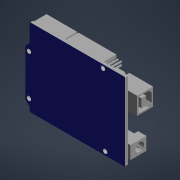
# Autodesk Inventor part: Arduino_Uno
Saved by Autodesk Inventor 2022 (Build 260153000, 153)
## iProperties
Created: 2016-11-21
Part Number: Arduino_Uno
Material: Genérico
Document SubType Name: Modeling
Designer: Dimitris
Density: 1 g/cm^3
Appearance: Por defecto
Author: Dimitris
Autodesk Inventor part; units mm, degrees
ref_plane "YZ Plane" through (0, 0, 0) normal (1, 0, 0) x (0, 1, 0)
ref_plane "XZ Plane" through (0, 0, 0) normal (0, 1, 0) x (-1, 0, 0)
sketch "Sketch1" plane through (0, 0, 0) normal (0, 1, 0) x (-1, 0, 0)
  line L0 (-3.5, 0) -> (-68, 0)
  line L1 (-68.5, -0.5) -> (-68.5, -53)
  line L2 (-68, -53.5) -> (-3.5, -53.5)
  line L3 (-3, -53) -> (-3, -50.5)
  line L4 (-3, -50.5) -> (-0.1464, -47.6464)
  line L5 (0, -15.7071) -> (0, -47.2929)
  line L6 (-3, -0.5) -> (-3, -12.5)
  line L7 (-0.1464, -15.3536) -> (-3, -12.5)
  arc A0 (-68.5, -53) -> (-68, -53.5) centre (-68, -53) ccw
  arc A1 (-68, 0) -> (-68.5, -0.5) centre (-68, -0.5) ccw
  arc A2 (-3.5, -53.5) -> (-3, -53) centre (-3.5, -53) ccw
  arc A3 (-0.1464, -47.6464) -> (0, -47.2929) centre (-0.5, -47.2929) ccw
  arc A4 (0, -15.7071) -> (-0.1464, -15.3536) centre (-0.5, -15.7071) ccw
  arc A5 (-3, -0.5) -> (-3.5, 0) centre (-3.5, -0.5) ccw
  point P0 (0, 0)
  point P1 (-68.5, -53.5)
  point P2 (-68.5, 0)
  point P3 (0, -47.5)
  point P4 (-3, -53.5)
  point P5 (0, -15.5)
  point P6 (-3, 0)
  dimension "d1" = 53.5
  dimension "d3" = 3
  dimension "d5" = 6
  dimension "d6" = 3
  dimension "d7" = 12.5
  dimension "d9" = 65.5
  dimension "d10" = 65.5
  dimension "d11" = 38
  dimension "d12" = 32
  dimension "d13" = 0.5
  constraints: 16 end point, 12 point on circle, 12 point on line, 12 tangent, 6 centre point, 5 equal radius, 3 parallel, 3 perpendicular, 1 horizontal
  measures "d1" distance of point (-68.5, -53.5) point (-68.5, 0)
  measures "d3" distance of point (-3, -53.5) L3.end
  measures "d5" distance from line of point (0, -47.5) L2
  measures "d6" distance between parallel lines of L5 L3
  measures "d7" distance of point (-3, 0) L6.end
  measures "d9" distance between parallel lines of L1 L6
  measures "d10" distance between parallel lines of L1 L3
  measures "d11" distance of L3.end L6.end
  measures "d12" distance of point (0, -15.5) point (0, -47.5)
  measures "d13" radius of A0
extrude "Extrusion1" add sketch "Sketch1" along normal blind 2
sketch "Sketch2" plane through (0, 2, 0) normal (0, 1, 0) x (1, 0, 0)
  line L0 (58.5, 1) -> (64.7, 1)
  line L1 (64.7, 1) -> (64.7, 7.2)
  line L2 (64.7, 7.2) -> (58.5, 7.2)
  line L3 (58.5, 7.2) -> (58.5, 1)
  point P0 (0, 0)
  dimension "d16" = 6.2
  dimension "d17" = 6.2
  constraints: 8 end point, 2 parallel, 1 horizontal, 1 perpendicular
  measures "d16" distance of L2.end L1.end
  measures "d17" distance of L1.end L0.end
extrude "Extrusion2" add sketch "Sketch2" along normal blind 2
sketch "Sketch3" plane through (0, 4, 0) normal (0, 1, 0) x (1, 0, 0)
  circle A0 centre (61.6, 4.1) radius 1.57
  point P0 (0, 0)
  dimension "d20" = 3.14
  constraints: 1 centre point
  measures "d20" diameter of A0
extrude "Extrusion3" add sketch "Sketch3" along normal blind 1.5
sketch "Sketch4" plane through (0, 2, 0) normal (0, 1, 0) x (1, 0, 0)
  line L0 (64.7, 7.2) -> (64.7, 1) projected
  line L1 (64.72, 1) -> (66.7, 1)
  line L2 (66.7, 1) -> (66.7, 1.8)
  line L3 (66.7, 1.8) -> (64.72, 1.8)
  line L4 (64.7, 1.8) -> (64.7, 1)
  line L5 (64.72, 3.7) -> (66.7, 3.7)
  line L6 (66.7, 3.7) -> (66.7, 4.5)
  line L7 (66.7, 4.5) -> (64.72, 4.5)
  line L8 (64.7, 4.5) -> (64.7, 3.7)
  line L9 (64.72, 7.2) -> (66.7, 7.2)
  line L10 (66.7, 7.2) -> (66.7, 6.4)
  line L11 (66.7, 6.4) -> (64.72, 6.4)
  line L12 (64.7, 6.4) -> (64.7, 7.2)
  line L13 (58.48, 7.2) -> (56.5, 7.2)
  line L14 (56.5, 7.2) -> (56.5, 6.4)
  line L15 (56.5, 6.4) -> (58.48, 6.4)
  line L16 (58.5, 6.4) -> (58.5, 7.2)
  line L17 (58.48, 1) -> (56.5, 1)
  line L18 (56.5, 1) -> (56.5, 1.8)
  line L19 (56.5, 1.8) -> (58.48, 1.8)
  line L20 (58.5, 1.8) -> (58.5, 1)
  line L21 (58.5, 1) -> (64.68, 1) construction
  line L22 (64.72, 6.4) -> (64.72, 7.2)
  line L23 (64.72, 1) -> (64.72, 1.8)
  line L24 (64.72, 3.7) -> (64.72, 4.5)
  line L25 (58.48, 1) -> (58.48, 1.8)
  line L26 (58.48, 6.4) -> (58.48, 7.2)
  point P0 (0, 0)
  dimension "d23" = 2
  dimension "d24" = 0.8
  dimension "d25" = 2
  dimension "d26" = 0.8
  dimension "d27" = 0.8
  dimension "d28" = 2
  dimension "d29" = 0.02
  dimension "d31" = 0.02
  constraints: 52 end point, 10 parallel, 8 perpendicular, 6 horizontal, 2 point on line
  measures "d23" distance of L4.start L2.end
  measures "d24" distance of L2.end L1.end
  measures "d25" distance of L8.start L6.end
  measures "d26" distance of L6.end L5.end
  measures "d27" distance of L9.end L10.end
  measures "d28" distance of L16.start L14.end
  measures "d29" distance of L17.start L20.end
  measures "d31" distance of L1.start L0.end
extrude "Extrusion4" add sketch "Sketch4" along normal blind 0.4
sketch "Sketch5" plane through (0, 2, 0) normal (0, 1, 0) x (1, 0, 0)
  line L0 (58.5, 9) -> (74.8, 9)
  line L1 (74.8, 9) -> (74.8, 21)
  line L2 (74.8, 21) -> (58.5, 21)
  line L3 (58.5, 21) -> (58.5, 9)
  line L4 (3.5, 0) -> (68, 0) projected
  point P0 (0, 0)
  dimension "d34" = 16.3
  dimension "d35" = 12
  dimension "d233" = 9
  constraints: 8 end point, 2 parallel, 1 horizontal, 1 perpendicular
  measures "d34" distance of L2.end L1.end
  measures "d35" distance of L1.end L0.end
  measures "d233" distance between parallel lines of L4 L0
extrude "Extrusion5" add sketch "Sketch5" along normal blind 11
sketch "Sketch6" plane through (74.8, 2, -9) normal (1, 0, 0) x (0, 0, -1)
  line L0 (0, 0) -> (12, 0) projected
  line L1 (12, 0) -> (12, 11) projected
  line L2 (11, 8) -> (11, 1)
  line L3 (11, 1) -> (1, 1)
  line L4 (1, 1) -> (1, 8)
  line L5 (1, 1) -> (1, 8)
  line L6 (9, 10) -> (11, 8)
  line L7 (9, 10) -> (3, 10)
  line L8 (3, 10) -> (1, 8)
  point P0 (-9, -2)
  dimension "d39" = 1
  dimension "d40" = 1
  dimension "d41" = 10
  dimension "d43" = 7
  dimension "d44" = 6
  constraints: 14 end point, 2 perpendicular
  measures "d39" distance between parallel lines of L0 L3
  measures "d40" distance between parallel lines of L1 L2
  measures "d41" distance of L2.end L3.end
  measures "d43" distance of L4.end L3.end
  measures "d44" distance of L6.start L7.end
extrude "Extrusion6" cut sketch "Sketch6" against normal blind 9
sketch "Sketch7" plane through (65.8, 2, -9) normal (1, 0, 0) x (0, 0, -1)
  line L0 (3, 3) -> (9, 3)
  line L1 (9, 3) -> (9, 6.2)
  line L2 (9, 6.2) -> (3, 6.2)
  line L3 (3, 6.2) -> (3, 3)
  point P0 (-9, -2)
  dimension "d47" = 6
  dimension "d48" = 3.2
  constraints: 8 end point, 2 parallel, 1 horizontal, 1 perpendicular
  measures "d47" distance of L2.end L1.end
  measures "d48" distance of L1.end L0.end
extrude "Extrusion7" add sketch "Sketch7" along normal blind 9
sketch "Boceto8" plane through (0, 2, 0) normal (0, 1, 0) x (1, 0, 0)
  circle A0 centre (2.4, 17.7) radius 1.5
  circle A1 centre (54.8, 51.1) radius 1.5
  circle A2 centre (53.3, 2.4) radius 1.5
  line L0 (3.5, 0) -> (68, 0) projected
  line L1 (68.5, 0.5) -> (68.5, 9) projected
  line L2 (0, 47.2929) -> (0, 15.7071) projected
  line L3 (53.3, 0.9) -> (48.8, 0.9) construction
  line L4 (54.8, 2.4) -> (54.8, 0) construction
  line L5 (54.8, 52.6) -> (48.6151, 52.6) construction
  line L6 (68, 53.5) -> (3.5, 53.5) construction
  line L7 (56.3, 51.1) -> (56.3, 48.9511) construction
  line L8 (68.5, 21) -> (68.5, 53) construction
  line L9 (0.9, 17.7) -> (0.9, 15.9278) construction
  circle A3 centre (2.4, 45.8) radius 1.5
  point P0 (0, 0)
  dimension "d52" = 3
  dimension "d53" = 3
  dimension "d54" = 3
  dimension "d79" = 2.4
  dimension "d80" = 15.2
  dimension "d220" = 17.7
  dimension "d221" = 2.4
  dimension "d222" = 2.4
  dimension "d223" = 13.7
  dimension "d227" = 3
  dimension "d228" = 2.4
  dimension "d229" = 7.7
  constraints: 10 end point, 4 point on circle, 4 tangent, 3 centre point, 3 vertical, 1 coincident, 1 horizontal, 1 horizontal alignment, 1 parallel, 1 perpendicular, 1 point on line, 2 other
  measures "d53" diameter of A1
  measures "d54" diameter of A2
  measures "d79" distance from line of L0 A2.centre
  measures "d80" distance from line of L1 A2.centre
  measures "d220" distance from line of point (2.4, 17.7) L0
  measures "d221" distance from line of L2 point (2.4, 17.7)
  measures "d222" distance from line of L6 A1.centre
  measures "d223" distance from line of L8 A1.centre
  measures "d227" diameter of A3
  measures "d228" distance from line of L2 A3.centre
  measures "d229" distance from line of L6 A3.centre
hole "Hole1" at (2.4, 2, -17.7) at (53.3, 2, -2.4) at (54.8, 2, -51.1) at (2.4, 2, -45.8) direction (0, -1, 0) diameter 3 end through all
sketch "Sketch9" plane through (0, 2, 0) normal (0, 1, 0) x (1, 0, 0)
  line L0 (56.5, 49.7) -> (70.1, 49.7)
  line L1 (70.1, 49.7) -> (70.1, 40.7)
  line L2 (70.1, 40.7) -> (56.5, 40.7)
  line L3 (56.5, 40.7) -> (56.5, 49.7)
  line L4 (68, 53.5) -> (3.5, 53.5) projected
  point P0 (0, 0)
  dimension "d62" = 13.6
  dimension "d63" = 9
  dimension "d232" = 3.8
  constraints: 8 end point, 2 parallel, 1 horizontal, 1 perpendicular
  measures "d62" distance of L1.end L2.end
  measures "d63" distance of L0.end L1.end
  measures "d232" distance between parallel lines of L4 L0
extrude "Extrusion8" add sketch "Sketch9" along normal blind 11
sketch "Sketch10" plane through (70.1, 2, -40.7) normal (1, 0, 0) x (0, 0, -1)
  circle A0 centre (4.5, 6.5) radius 3
  point P0 (-40.7, -2)
  dimension "d66" = 6
  constraints: 1 centre point
  measures "d66" diameter of A0
extrude "Extrusion9" cut sketch "Sketch10" against normal blind 8
sketch "Sketch11" plane through (56.5, 2, -49.7) normal (-1, 0, 0) x (0, 0, 1)
  line L0 (9, 0) -> (0, 0) projected
  line L1 (9, 0) -> (9, 11) projected
  line L2 (0, 11) -> (9, 11) projected
  line L3 (0, 0) -> (0, 11) projected
  arc A0 (9, 6.5) -> (0, 6.5) centre (4.5, 6.5) ccw
  line L4 (0, 6.5) -> (0, 11)
  line L5 (9, 11) -> (0, 11)
  line L6 (9, 11) -> (9, 6.5)
  point P0 (49.7, -2)
  constraints: 6 end point, 2 collinear, 2 point on circle, 2 point on line, 2 tangent, 1 centre point
extrude "Extrusion10" cut sketch "Sketch11" against normal blind 8 contours A0 L2 L1 | L3 L2 A0
sketch "Sketch12" plane through (62.1, 8.5, -45.2) normal (1, 0, 0) x (0, 0, -1)
  circle A0 centre (0, 0) radius 3 projected
  circle A1 centre (0, 0) radius 0.6
  point P0 (-45.2, -8.5)
  dimension "d71" = 1.2
  constraints: 1 centre point, 1 coincident
  measures "d71" diameter of A1
extrude "Extrusion11" add sketch "Sketch12" along normal blind 8 contours A1
sketch "Sketch13" plane through (0, 2, 0) normal (0, 1, 0) x (1, 0, 0)
  arc A0 (3, 0.5) -> (3.5, 0) centre (3.5, 0.5) ccw projected
  line L0 (3.5, 0.5) -> (24.5, 0.5)
  line L1 (24.5, 0.5) -> (24.5, 3)
  line L2 (24.5, 3) -> (3.5, 3)
  line L3 (3.5, 3) -> (3.5, 0.5)
  line L4 (25.45, 0.5) -> (51.45, 0.5)
  line L5 (51.45, 0.5) -> (51.45, 3)
  line L6 (51.45, 3) -> (25.45, 3)
  line L7 (25.45, 3) -> (25.45, 0.5)
  point P0 (0, 0)
  dimension "d74" = 21
  dimension "d75" = 2.5
  dimension "d76" = 26
  dimension "d230" = 0.95
  constraints: 16 end point, 4 parallel, 2 horizontal, 2 perpendicular
  measures "d74" distance of L2.end L1.end
  measures "d75" distance of L1.end L0.end
  measures "d76" distance of L6.end L5.end
  measures "d230" distance between parallel lines of L1 L7
extrude "Extrusion12" add sketch "Sketch13" along normal blind 9
sketch "Sketch14" plane through (0, 11, 0) normal (0, 1, 0) x (1, 0, 0)
  line L0 (3.5, 0.5) -> (24.5, 0.5) projected
  line L1 (23.75, 2.25) -> (23.75, 1.25)
  line L2 (4.25, 1.25) -> (4.25, 2.25)
  line L3 (4.25, 1.25) -> (5.25, 1.25)
  line L4 (5.25, 1.25) -> (5.25, 2.25)
  line L5 (5.25, 2.25) -> (4.25, 2.25)
  line L6 (4.25, 2.25) -> (4.25, 1.25)
  line L7 (6.9, 1.25) -> (7.9, 1.25)
  line L8 (7.9, 1.25) -> (7.9, 2.25)
  line L9 (7.9, 2.25) -> (6.9, 2.25)
  line L10 (6.9, 2.25) -> (6.9, 1.25)
  line L11 (9.55, 1.25) -> (10.55, 1.25)
  line L12 (10.55, 1.25) -> (10.55, 2.25)
  line L13 (10.55, 2.25) -> (9.55, 2.25)
  line L14 (9.55, 2.25) -> (9.55, 1.25)
  line L15 (12.2, 1.25) -> (13.2, 1.25)
  line L16 (13.2, 1.25) -> (13.2, 2.25)
  line L17 (13.2, 2.25) -> (12.2, 2.25)
  line L18 (12.2, 2.25) -> (12.2, 1.25)
  line L19 (14.85, 1.25) -> (15.85, 1.25)
  line L20 (15.85, 1.25) -> (15.85, 2.25)
  line L21 (15.85, 2.25) -> (14.85, 2.25)
  line L22 (14.85, 2.25) -> (14.85, 1.25)
  line L23 (17.5, 1.25) -> (18.5, 1.25)
  line L24 (18.5, 1.25) -> (18.5, 2.25)
  line L25 (18.5, 2.25) -> (17.5, 2.25)
  line L26 (17.5, 2.25) -> (17.5, 1.25)
  line L27 (20.15, 1.25) -> (21.15, 1.25)
  line L28 (21.15, 1.25) -> (21.15, 2.25)
  line L29 (21.15, 2.25) -> (20.15, 2.25)
  line L30 (20.15, 2.25) -> (20.15, 1.25)
  line L31 (22.8, 1.25) -> (23.8, 1.25)
  line L32 (23.8, 1.25) -> (23.8, 2.25)
  line L33 (23.8, 2.25) -> (22.8, 2.25)
  line L34 (22.8, 2.25) -> (22.8, 1.25)
  line L35 (4.25, 2.25) -> (5.25, 2.25)
  line L36 (5.25, 1.25) -> (4.25, 1.25)
  line L37 (6.9, 2.25) -> (7.9, 2.25)
  line L38 (7.9, 1.25) -> (6.9, 1.25)
  line L39 (9.55, 2.25) -> (10.55, 2.25)
  line L40 (10.55, 1.25) -> (9.55, 1.25)
  line L41 (12.2, 2.25) -> (13.2, 2.25)
  line L42 (13.2, 1.25) -> (12.2, 1.25)
  line L43 (14.85, 2.25) -> (15.85, 2.25)
  line L44 (15.85, 1.25) -> (14.85, 1.25)
  line L45 (17.5, 2.25) -> (18.5, 2.25)
  line L46 (18.5, 1.25) -> (17.5, 1.25)
  line L47 (20.15, 2.25) -> (21.15, 2.25)
  line L48 (22.8, 2.25) -> (23.75, 2.25)
  line L49 (23.75, 1.25) -> (22.8, 1.25)
  line L50 (21.15, 1.25) -> (20.15, 1.25)
  point P0 (0, 0)
  dimension "d82" = 1
  dimension "d85" = 2.65
  constraints: 100 end point, 2 horizontal, 2 parallel, 1 perpendicular, 56 other
  measures "d82" distance of L5.end L4.end
  measures "d85" distance of L3.end L8.start
extrude "Extrusion13" cut sketch "Sketch14" against normal blind 1 contours L1 L31 L34 L33 | L2 L5 L4 L3 | L10 L9 L8 L7 | L14 L13 L12 L11 | L18 L17 L16 L15 | L22 L21 L20 L19 | L26 L25 L24 L23 | L30 L29 L28 L27
sketch "Sketch15" plane through (0, 11, 0) normal (0, 1, 0) x (1, 0, 0)
  line L0 (25.45, 0.5) -> (51.45, 0.5) projected
  line L1 (26.75, 1.25) -> (26.75, 2.25)
  line L2 (26.75, 2.25) -> (27.75, 2.25)
  line L3 (27.75, 2.25) -> (27.75, 1.25)
  line L4 (27.75, 1.25) -> (26.75, 1.25)
  line L5 (26.75, 1.25) -> (26.75, 2.25)
  line L6 (29.36, 2.25) -> (30.36, 2.25)
  line L7 (30.36, 2.25) -> (30.36, 1.25)
  line L8 (30.36, 1.25) -> (29.36, 1.25)
  line L9 (29.36, 1.25) -> (29.36, 2.25)
  line L10 (31.97, 2.25) -> (32.97, 2.25)
  line L11 (32.97, 2.25) -> (32.97, 1.25)
  line L12 (32.97, 1.25) -> (31.97, 1.25)
  line L13 (31.97, 1.25) -> (31.97, 2.25)
  line L14 (34.58, 2.25) -> (35.58, 2.25)
  line L15 (35.58, 2.25) -> (35.58, 1.25)
  line L16 (35.58, 1.25) -> (34.58, 1.25)
  line L17 (34.58, 1.25) -> (34.58, 2.25)
  line L18 (37.19, 2.25) -> (38.19, 2.25)
  line L19 (38.19, 2.25) -> (38.19, 1.25)
  line L20 (38.19, 1.25) -> (37.19, 1.25)
  line L21 (37.19, 1.25) -> (37.19, 2.25)
  line L22 (39.8, 2.25) -> (40.8, 2.25)
  line L23 (40.8, 2.25) -> (40.8, 1.25)
  line L24 (40.8, 1.25) -> (39.8, 1.25)
  line L25 (39.8, 1.25) -> (39.8, 2.25)
  line L26 (42.41, 2.25) -> (43.41, 2.25)
  line L27 (43.41, 2.25) -> (43.41, 1.25)
  line L28 (43.41, 1.25) -> (42.41, 1.25)
  line L29 (42.41, 1.25) -> (42.41, 2.25)
  line L30 (45.02, 2.25) -> (46.02, 2.25)
  line L31 (46.02, 2.25) -> (46.02, 1.25)
  line L32 (46.02, 1.25) -> (45.02, 1.25)
  line L33 (45.02, 1.25) -> (45.02, 2.25)
  line L34 (47.63, 2.25) -> (48.63, 2.25)
  line L35 (48.63, 2.25) -> (48.63, 1.25)
  line L36 (48.63, 1.25) -> (47.63, 1.25)
  line L37 (47.63, 1.25) -> (47.63, 2.25)
  line L38 (50.24, 2.25) -> (51.24, 2.25)
  line L39 (51.24, 2.25) -> (51.24, 1.25)
  line L40 (51.24, 1.25) -> (50.24, 1.25)
  line L41 (50.24, 1.25) -> (50.24, 2.25)
  line L42 (50.24, 2.25) -> (51.24, 2.25)
  line L43 (51.24, 1.25) -> (50.24, 1.25)
  line L44 (47.63, 2.25) -> (48.63, 2.25)
  line L45 (48.63, 1.25) -> (47.63, 1.25)
  line L46 (45.02, 2.25) -> (46.02, 2.25)
  line L47 (46.02, 1.25) -> (45.02, 1.25)
  line L48 (43.41, 1.25) -> (42.41, 1.25)
  line L49 (42.41, 2.25) -> (43.41, 2.25)
  line L50 (40.8, 1.25) -> (39.8, 1.25)
  line L51 (39.8, 2.25) -> (40.8, 2.25)
  line L52 (38.19, 1.25) -> (37.19, 1.25)
  line L53 (37.19, 2.25) -> (38.19, 2.25)
  line L54 (34.58, 2.25) -> (35.58, 2.25)
  line L55 (35.58, 1.25) -> (34.58, 1.25)
  line L56 (32.97, 1.25) -> (31.97, 1.25)
  line L57 (31.97, 2.25) -> (32.97, 2.25)
  line L58 (26.75, 2.25) -> (27.75, 2.25)
  line L59 (29.36, 2.25) -> (30.36, 2.25)
  line L60 (30.36, 1.25) -> (29.36, 1.25)
  line L61 (27.75, 1.25) -> (26.75, 1.25)
  point P0 (0, 0)
  dimension "d93" = 1
  dimension "d96" = 2.61
  constraints: 122 end point, 2 horizontal, 2 parallel, 1 perpendicular, 72 other
  measures "d93" distance of L3.end L4.end
  measures "d96" distance of L2.end L7.start
extrude "Extrusion14" cut sketch "Sketch15" against normal blind 1
sketch "Sketch16" plane through (0, 2, 0) normal (0, 1, 0) x (1, 0, 0)
  line L0 (5.05, 52.5) -> (20.35, 52.5)
  line L1 (20.35, 52.5) -> (20.35, 50)
  line L2 (20.35, 50) -> (5.05, 50)
  line L3 (5.05, 50) -> (5.05, 52.5)
  line L4 (22.3, 52.5) -> (43.3, 52.5)
  line L5 (43.3, 52.5) -> (43.3, 50)
  line L6 (43.3, 50) -> (22.3, 50)
  line L7 (22.3, 50) -> (22.3, 52.5)
  point P0 (0, 0)
  dimension "d103" = 15.3
  dimension "d104" = 2.5
  dimension "d105" = 21
  dimension "d231" = 1.95
  constraints: 16 end point, 4 parallel, 2 horizontal, 2 perpendicular
  measures "d103" distance of L1.end L2.end
  measures "d104" distance of L0.end L1.end
  measures "d105" distance of L5.end L6.end
  measures "d231" distance between parallel lines of L1 L7
extrude "Extrusion15" add sketch "Sketch16" along normal blind 9
sketch "Sketch17" plane through (0, 11, 0) normal (0, 1, 0) x (1, 0, 0)
  line L0 (22.3, 52.5) -> (22.3, 50) projected
  line L1 (22.3, 50) -> (43.3, 50) projected
  line L2 (43.3, 50) -> (43.3, 52.5) projected
  line L3 (42.55, 51.75) -> (42.55, 50.75)
  line L4 (42.55, 50.75) -> (23.05, 50.75)
  line L5 (23.05, 50.75) -> (23.05, 51.75)
  line L6 (23.05, 51.75) -> (24.05, 51.75)
  line L7 (24.05, 51.75) -> (24.05, 50.75)
  line L8 (24.05, 50.75) -> (23.05, 50.75)
  line L9 (23.05, 50.75) -> (23.05, 51.75)
  line L10 (25.7, 51.75) -> (26.7, 51.75)
  line L11 (26.7, 51.75) -> (26.7, 50.75)
  line L12 (26.7, 50.75) -> (25.7, 50.75)
  line L13 (25.7, 50.75) -> (25.7, 51.75)
  line L14 (28.35, 51.75) -> (29.35, 51.75)
  line L15 (29.35, 51.75) -> (29.35, 50.75)
  line L16 (29.35, 50.75) -> (28.35, 50.75)
  line L17 (28.35, 50.75) -> (28.35, 51.75)
  line L18 (31, 51.75) -> (32, 51.75)
  line L19 (32, 51.75) -> (32, 50.75)
  line L20 (32, 50.75) -> (31, 50.75)
  line L21 (31, 50.75) -> (31, 51.75)
  line L22 (33.65, 51.75) -> (34.65, 51.75)
  line L23 (34.65, 51.75) -> (34.65, 50.75)
  line L24 (34.65, 50.75) -> (33.65, 50.75)
  line L25 (33.65, 50.75) -> (33.65, 51.75)
  line L26 (36.3, 51.75) -> (37.3, 51.75)
  line L27 (37.3, 51.75) -> (37.3, 50.75)
  line L28 (37.3, 50.75) -> (36.3, 50.75)
  line L29 (36.3, 50.75) -> (36.3, 51.75)
  line L30 (38.95, 51.75) -> (39.95, 51.75)
  line L31 (39.95, 51.75) -> (39.95, 50.75)
  line L32 (39.95, 50.75) -> (38.95, 50.75)
  line L33 (38.95, 50.75) -> (38.95, 51.75)
  line L34 (41.6, 51.75) -> (42.6, 51.75)
  line L35 (42.6, 51.75) -> (42.6, 50.75)
  line L36 (42.6, 50.75) -> (41.6, 50.75)
  line L37 (41.6, 50.75) -> (41.6, 51.75)
  line L38 (41.6, 51.75) -> (42.55, 51.75)
  line L39 (38.95, 51.75) -> (39.95, 51.75)
  line L40 (36.3, 51.75) -> (37.3, 51.75)
  line L41 (33.65, 51.75) -> (34.65, 51.75)
  line L42 (31, 51.75) -> (32, 51.75)
  line L43 (28.35, 51.75) -> (29.35, 51.75)
  line L44 (23.05, 51.75) -> (24.05, 51.75)
  line L45 (25.7, 51.75) -> (26.7, 51.75)
  point P0 (0, 0)
  dimension "d109" = 1
  dimension "d112" = 2.65
  constraints: 86 end point, 2 horizontal, 2 parallel, 1 perpendicular, 1 point on line, 58 other
  measures "d109" distance of L7.end L8.end
  measures "d112" distance of L7.end L12.start
extrude "Extrusion16" cut sketch "Sketch17" against normal blind 1
sketch "Sketch18" plane through (0, 11, 0) normal (0, 1, 0) x (1, 0, 0)
  line L0 (5.05, 52.5) -> (5.05, 50) projected
  line L1 (5.05, 50) -> (20.35, 50) projected
  line L2 (19.55, 50.75) -> (5.8, 50.75)
  line L3 (5.8, 50.75) -> (5.8, 51.75)
  line L4 (5.8, 51.75) -> (6.8, 51.75)
  line L5 (6.8, 51.75) -> (6.8, 50.75)
  line L6 (6.8, 50.75) -> (5.8, 50.75)
  line L7 (5.8, 50.75) -> (5.8, 51.75)
  line L8 (8.4, 51.75) -> (9.4, 51.75)
  line L9 (9.4, 51.75) -> (9.4, 50.75)
  line L10 (9.4, 50.75) -> (8.4, 50.75)
  line L11 (8.4, 50.75) -> (8.4, 51.75)
  line L12 (11, 51.75) -> (12, 51.75)
  line L13 (12, 51.75) -> (12, 50.75)
  line L14 (12, 50.75) -> (11, 50.75)
  line L15 (11, 50.75) -> (11, 51.75)
  line L16 (13.6, 51.75) -> (14.6, 51.75)
  line L17 (14.6, 51.75) -> (14.6, 50.75)
  line L18 (14.6, 50.75) -> (13.6, 50.75)
  line L19 (13.6, 50.75) -> (13.6, 51.75)
  line L20 (16.2, 51.75) -> (17.2, 51.75)
  line L21 (17.2, 51.75) -> (17.2, 50.75)
  line L22 (17.2, 50.75) -> (16.2, 50.75)
  line L23 (16.2, 50.75) -> (16.2, 51.75)
  line L24 (18.8, 51.75) -> (19.8, 51.75)
  line L25 (19.8, 51.75) -> (19.8, 50.75)
  line L26 (19.8, 50.75) -> (18.8, 50.75)
  line L27 (18.8, 50.75) -> (18.8, 51.75)
  line L28 (18.8, 51.75) -> (19.6, 51.75)
  line L29 (16.2, 51.75) -> (17.2, 51.75)
  line L30 (13.6, 51.75) -> (14.6, 51.75)
  line L31 (11, 51.75) -> (12, 51.75)
  line L32 (5.8, 51.75) -> (6.8, 51.75)
  line L33 (8.4, 51.75) -> (9.4, 51.75)
  point P0 (0, 0)
  dimension "d120" = 1
  dimension "d123" = 2.6
  constraints: 64 end point, 2 horizontal, 2 parallel, 1 perpendicular, 1 point on line, 41 other
  measures "d120" distance of L5.end L6.end
  measures "d123" distance of L3.end L8.start
extrude "Extrusion17" cut sketch "Sketch18" against normal blind 1
sketch "Sketch19" plane through (0, 2, 0) normal (0, 1, 0) x (1, 0, 0)
  line L0 (4.5, 42) -> (40.1, 42)
  line L1 (40.1, 42) -> (40.1, 32)
  line L2 (40.1, 32) -> (4.5, 32)
  line L3 (4.5, 32) -> (4.5, 42)
  point P0 (0, 0)
  dimension "d130" = 35.6
  dimension "d131" = 10
  constraints: 8 end point, 2 parallel, 1 horizontal, 1 perpendicular
  measures "d130" distance of L1.end L2.end
  measures "d131" distance of L0.end L1.end
extrude "Extrusion18" add sketch "Sketch19" along normal blind 4
sketch "Sketch20" plane through (0, 6, 0) normal (0, 1, 0) x (1, 0, 0)
  line L0 (4.6, 32.5) -> (40, 32.5)
  line L1 (40, 32.5) -> (40, 41.5)
  line L2 (40, 41.5) -> (4.6, 41.5)
  line L3 (4.6, 41.5) -> (4.6, 32.5)
  point P0 (0, 0)
  dimension "d134" = 35.4
  dimension "d135" = 9
  constraints: 8 end point, 2 parallel, 1 horizontal, 1 perpendicular
  measures "d134" distance of L2.end L1.end
  measures "d135" distance of L1.end L0.end
extrude "Extrusion19" add sketch "Sketch20" along normal blind 3
chamfer "Chamfer1" distance 0.2 angle 45 8 edges at (22.3, 9, -32.5) (4.6, 9, -37) (22.3, 9, -41.5) (40, 9, -37) (40, 7.5, -32.5) (40, 7.5, -41.5) (4.6, 7.5, -32.5) (4.6, 7.5, -41.5)
sketch "Sketch21" plane through (4.8, 6, -32.5) normal (0, 0, 1) x (1, 0, 0)
  line L0 (35, 0) -> (0, 0) projected
  line L1 (0.5, 0) -> (2, 0)
  line L2 (2, 0) -> (2, 2.5)
  line L3 (2, 2.5) -> (0.5, 2.5)
  line L4 (0.5, 2.5) -> (0.5, 0)
  point P0 (-4.8, -6)
  dimension "d141" = 1.5
  dimension "d142" = 2.5
  constraints: 8 end point, 2 parallel, 1 horizontal, 1 perpendicular, 1 point on line
  measures "d141" distance of L3.end L2.end
  measures "d142" distance of L2.end L1.end
extrude "Extrusion20" add sketch "Sketch21" along normal blind 0.3
pattern_linear "Rectangular Pattern1" count 14 spacing 2.48 along (1, 0, 0) of "Extrusion20"
ref_plane "Work Plane1" through (4.8, 8.8, -37) normal (0, 0, 1) x (1, 0, 0)
mirror "Mirror1" about plane through (4.8, 8.8, -37) normal (0, 0, 1) of "Extrusion20", "Rectangular Pattern1"
sketch "Sketch22" plane through (0, 2, 0) normal (0, 1, 0) x (1, 0, 0)
  line L0 (0, 47.2929) -> (0, 15.7071) projected
  line L1 (3.5, 0) -> (68, 0) projected
  circle A0 centre (43, 45) radius 3.1
  circle A1 centre (49.3, 45) radius 3.1
  point P0 (0, 0)
  dimension "d27" = 0.8
  dimension "d148" = 6.2
  dimension "d149" = 6.2
  dimension "d150" = 6.3
  dimension "d151" = 45
  dimension "d152" = 43
  constraints: 2 centre point
  measures "d148" diameter of A0
  measures "d149" diameter of A1
  measures "d150" distance of A1.centre A0.centre
  measures "d151" distance from line of L1 A0.centre
  measures "d152" distance from line of L0 A0.centre
extrude "Extrusion21" add sketch "Sketch22" along normal blind 5
sketch "Sketch23" plane through (0, 2, 0) normal (0, 1, 0) x (1, 0, 0)
  line L0 (1.75, 20) -> (6.75, 20)
  line L1 (6.75, 20) -> (6.75, 27.5)
  line L2 (6.75, 27.5) -> (1.75, 27.5)
  line L3 (1.75, 27.5) -> (1.75, 20)
  line L4 (53.5, 4.5) -> (46, 4.5)
  line L5 (46, 4.5) -> (46, 9.5)
  line L6 (46, 9.5) -> (53.5, 9.5)
  line L7 (53.5, 9.5) -> (53.5, 4.5)
  point P0 (0, 0)
  dimension "d155" = 5
  dimension "d156" = 7.5
  dimension "d157" = 7.5
  dimension "d158" = 5
  constraints: 16 end point, 4 parallel, 2 horizontal, 2 perpendicular
  measures "d155" distance of L2.end L1.end
  measures "d156" distance of L1.end L0.end
  measures "d157" distance of L5.end L6.end
  measures "d158" distance of L4.end L5.end
extrude "Extrusion22" add sketch "Sketch23" along normal blind 2
sketch "Sketch24" plane through (0, 2, 0) normal (0, 1, 0) x (1, 0, 0)
  line L0 (46, 20) -> (51, 20)
  line L1 (51, 20) -> (51, 15)
  line L2 (51, 15) -> (46, 15)
  line L3 (46, 15) -> (46, 20)
  point P0 (0, 0)
  dimension "d161" = 5
  dimension "d162" = 5
  constraints: 8 end point, 2 parallel, 1 horizontal, 1 perpendicular
  measures "d161" distance of L1.end L2.end
  measures "d162" distance of L0.end L1.end
extrude "Extrusion23" add sketch "Sketch24" along normal blind 1
sketch "Sketch25" plane through (0, 2, 0) normal (0, 1, 0) x (1, 0, 0)
  line L0 (45.1504, 52.5) -> (50.1504, 52.5)
  line L1 (50.1504, 52.5) -> (50.1504, 50)
  line L2 (50.1504, 50) -> (45.1504, 50)
  line L3 (45.1504, 50) -> (45.1504, 52.5)
  point P0 (0, 0)
  dimension "d165" = 5
  constraints: 8 end point, 2 parallel, 1 horizontal, 1 perpendicular
  measures "d165" distance of L1.end L2.end
extrude "Extrusion24" add sketch "Sketch25" along normal blind 0.5
sketch "Sketch26" plane through (0, 2.5, 0) normal (0, 1, 0) x (1, 0, 0)
  line L0 (50.1504, 52.5) -> (45.1504, 52.5) projected
  line L1 (45.1504, 50) -> (50.1504, 50) projected
  line L2 (46.15, 52.5) -> (49.15, 52.5)
  line L3 (49.15, 52.5) -> (49.15, 50)
  line L4 (49.15, 50) -> (46.15, 50)
  line L5 (46.15, 50) -> (46.15, 52.5)
  point P0 (0, 0)
  dimension "d168" = 3
  constraints: 8 end point, 2 parallel, 2 point on line, 1 horizontal, 1 perpendicular
  measures "d168" distance of L3.end L4.end
extrude "Extrusion25" add sketch "Sketch26" along normal blind 1
sketch "Sketch27" plane through (0, 2, 0) normal (0, 1, 0) x (1, 0, 0)
  line L0 (63.5, 38.5) -> (61.5, 38.5)
  line L1 (61.5, 38.5) -> (61.5, 33.5)
  line L2 (61.5, 33.5) -> (63.5, 33.5)
  line L3 (63.5, 33.5) -> (63.5, 38.5)
  point P0 (0, 0)
  dimension "d171" = 2
  dimension "d172" = 5
  constraints: 8 end point, 2 parallel, 1 horizontal, 1 perpendicular
  measures "d171" distance of L2.end L1.end
  measures "d172" distance of L1.end L0.end
extrude "Extrusion26" add sketch "Sketch27" along normal blind 1
sketch "Sketch28" plane through (0, 4, 0) normal (0, 1, 0) x (1, 0, 0)
  line L0 (1.75, 20) -> (6.75, 20) projected
  line L1 (6.75, 27.5) -> (1.75, 27.5) projected
  line L2 (1.75, 27.5) -> (1.75, 20) projected
  line L3 (2.75, 26.5) -> (5.75, 26.5)
  line L4 (5.75, 21) -> (2.75, 21)
  line L5 (2.75, 21) -> (2.75, 26.5)
  line L6 (2.75, 26.5) -> (3.55, 26.5)
  line L7 (3.55, 26.5) -> (3.55, 25.7)
  line L8 (3.55, 25.7) -> (2.75, 25.7)
  line L9 (2.75, 25.7) -> (2.75, 26.5)
  line L10 (2.75, 24.15) -> (3.55, 24.15)
  line L11 (3.55, 24.15) -> (3.55, 23.35)
  line L12 (3.55, 23.35) -> (2.75, 23.35)
  line L13 (2.75, 23.35) -> (2.75, 24.15)
  line L14 (2.75, 21.8) -> (3.55, 21.8)
  line L15 (3.55, 21.8) -> (3.55, 21)
  line L16 (3.55, 21) -> (2.75, 21)
  line L17 (2.75, 21) -> (2.75, 21.8)
  line L18 (4.95, 26.5) -> (5.75, 26.5)
  line L19 (5.75, 26.5) -> (5.75, 25.7)
  line L20 (5.75, 25.7) -> (4.95, 25.7)
  line L21 (4.95, 25.7) -> (4.95, 26.5)
  line L22 (4.95, 24.15) -> (5.75, 24.15)
  line L23 (5.75, 24.15) -> (5.75, 23.35)
  line L24 (5.75, 23.35) -> (4.95, 23.35)
  line L25 (4.95, 23.35) -> (4.95, 24.15)
  line L26 (4.95, 21.8) -> (5.75, 21.8)
  line L27 (5.75, 21.8) -> (5.75, 21)
  line L28 (5.75, 21) -> (4.95, 21)
  line L29 (4.95, 21) -> (4.95, 21.8)
  line L30 (5.75, 26.5) -> (5.75, 25.7)
  line L31 (5.75, 24.15) -> (5.75, 23.35)
  line L32 (5.75, 21.8) -> (5.75, 21)
  point P0 (0, 0)
  dimension "d175" = 1
  dimension "d180" = 2.35
  dimension "d183" = 2.2
  constraints: 60 end point, 2 horizontal, 2 parallel, 1 perpendicular, 1 vertical, 41 other
  measures "d175" distance between parallel lines of L1 L3
  measures "d180" distance of L7.end L12.start
  measures "d183" distance of L7.end L20.start
extrude "Extrusion27" add sketch "Sketch28" along normal blind 10
sketch "Sketch29" plane through (0, 2, 0) normal (0, 1, 0) x (1, 0, 0)
  line L0 (43.3, 24.4545) -> (53.3, 24.4545)
  line L1 (53.3, 27.9545) -> (43.3, 27.9545)
  arc A0 (43.3, 27.9545) -> (43.3, 24.4545) centre (43.3, 26.2045) ccw
  arc A1 (53.3, 24.4545) -> (53.3, 27.9545) centre (53.3, 26.2045) ccw
  point P0 (0, 0)
  dimension "d188" = 10
  dimension "d189" = 3.5
  constraints: 4 end point, 4 point on circle, 2 centre point, 1 horizontal, 1 parallel
  measures "d188" distance of L1.end L1.start
  measures "d189" distance of L1.start L0.end
extrude "Extrusion28" add sketch "Sketch29" along normal blind 4
fillet "Fillet1" radius 0.5 4 edges at (55.05, 6, -26.2045) (48.3, 6, -27.9545) (41.55, 6, -26.2045) (48.3, 6, -24.4545)
sketch "Sketch30" plane through (0, 4, 0) normal (0, 1, 0) x (1, 0, 0)
  line L0 (46, 4.5) -> (53.5, 4.5) projected
  line L1 (53.5, 4.5) -> (53.5, 9.5) projected
  line L2 (53.5, 9.5) -> (46, 9.5) projected
  line L3 (46, 9.5) -> (46, 4.5) projected
  line L4 (47, 8.5) -> (52.5, 8.5)
  line L5 (52.5, 8.5) -> (52.5, 5.5)
  line L6 (52.5, 5.5) -> (47, 5.5)
  line L7 (47, 5.5) -> (47, 8.5)
  line L8 (47, 5.5) -> (47.8, 5.5)
  line L9 (47.8, 5.5) -> (47.8, 6.3)
  line L10 (47.8, 6.3) -> (47, 6.3)
  line L11 (47, 6.3) -> (47, 5.5)
  line L12 (49.35, 5.5) -> (50.15, 5.5)
  line L13 (50.15, 5.5) -> (50.15, 6.3)
  line L14 (50.15, 6.3) -> (49.35, 6.3)
  line L15 (49.35, 6.3) -> (49.35, 5.5)
  line L16 (51.7, 5.5) -> (52.5, 5.5)
  line L17 (52.5, 5.5) -> (52.5, 6.3)
  line L18 (52.5, 6.3) -> (51.7, 6.3)
  line L19 (51.7, 6.3) -> (51.7, 5.5)
  line L20 (47, 7.7) -> (47.8, 7.7)
  line L21 (47.8, 7.7) -> (47.8, 8.5)
  line L22 (47.8, 8.5) -> (47, 8.5)
  line L23 (47, 8.5) -> (47, 7.7)
  line L24 (49.35, 7.7) -> (50.15, 7.7)
  line L25 (50.15, 7.7) -> (50.15, 8.5)
  line L26 (50.15, 8.5) -> (49.35, 8.5)
  line L27 (49.35, 8.5) -> (49.35, 7.7)
  line L28 (51.7, 7.7) -> (52.5, 7.7)
  line L29 (52.5, 7.7) -> (52.5, 8.5)
  line L30 (52.5, 8.5) -> (51.7, 8.5)
  line L31 (51.7, 8.5) -> (51.7, 7.7)
  point P0 (0, 0)
  dimension "d193" = 1
  dimension "d194" = 0.8
  dimension "d195" = 0.8
  dimension "d198" = 2.35
  dimension "d201" = 2.2
  constraints: 56 end point, 2 horizontal, 2 parallel, 1 perpendicular, 1 vertical, 43 other
  measures "d193" distance between parallel lines of L2 L4
  measures "d194" distance of L10.end L9.end
  measures "d195" distance of L9.end L8.end
  measures "d198" distance of L8.end L13.start
  measures "d201" distance of L8.end L21.start
extrude "Extrusion29" add sketch "Sketch30" along normal blind 10 contours L4 L21 L20 L7 | L4 L25 L24 L27 | L10 L9 L6 L7 | L4 L5 L28 L31 | L15 L14 L13 L6 | L5 L6 L19 L18
sketch "Sketch31" plane through (0, 2, 0) normal (0, 1, 0) x (1, 0, 0)
  line L0 (39, 11) -> (35.75, 11)
  line L1 (35.75, 11) -> (35.75, 12.5)
  line L2 (35.75, 12.5) -> (39, 12.5)
  line L3 (39, 12.5) -> (39, 11)
  line L4 (39, 17.2071) -> (35.75, 17.2071)
  line L5 (35.75, 17.2071) -> (35.75, 18.7071)
  line L6 (35.75, 18.7071) -> (39, 18.7071)
  line L7 (39, 18.7071) -> (39, 17.2071)
  line L8 (39, 20) -> (35.75, 20)
  line L9 (35.75, 20) -> (35.75, 21.5)
  line L10 (35.75, 21.5) -> (39, 21.5)
  line L11 (39, 21.5) -> (39, 20)
  point P0 (0, 0)
  dimension "d206" = 1.5
  dimension "d207" = 3.25
  dimension "d208" = 3.25
  dimension "d209" = 1.5
  dimension "d210" = 1.5
  constraints: 24 end point, 6 parallel, 3 horizontal, 3 perpendicular
  measures "d206" distance of L0.end L1.end
  measures "d207" distance of L0.start L0.end
  measures "d208" distance of L5.end L6.end
  measures "d209" distance of L4.end L5.end
  measures "d210" distance of L8.end L9.end
extrude "Extrusion30" add sketch "Sketch31" along normal blind 0.2
sketch "Sketch32" plane through (0, 2, 0) normal (0, 1, 0) x (1, 0, 0)
  line L0 (35.75, 17.2071) -> (35.75, 18.7071) projected
  line L1 (39, 18.7071) -> (39, 17.2071) projected
  line L2 (35.75, 11) -> (35.75, 12.5) projected
  line L3 (39, 12.5) -> (39, 11) projected
  line L4 (35.75, 20) -> (35.75, 21.5) projected
  line L5 (39, 21.5) -> (39, 20) projected
  line L6 (35.75, 21.3) -> (34.95, 21.3)
  line L7 (34.95, 21.3) -> (34.95, 20.2)
  line L8 (34.95, 20.2) -> (35.75, 20.2)
  line L9 (35.75, 20.2) -> (35.75, 21.3)
  line L10 (39, 21.3) -> (39.8, 21.3)
  line L11 (39.8, 21.3) -> (39.8, 20.2)
  line L12 (39.8, 20.2) -> (39, 20.2)
  line L13 (39, 20.2) -> (39, 21.3)
  line L14 (35.75, 18.407) -> (34.8304, 18.407)
  line L15 (34.8304, 18.407) -> (34.8304, 17.307)
  line L16 (34.8304, 17.307) -> (35.75, 17.307)
  line L17 (35.75, 17.307) -> (35.75, 18.407)
  line L18 (39, 18.407) -> (39.8, 18.407)
  line L19 (39.8, 18.407) -> (39.8, 17.307)
  line L20 (39.8, 17.307) -> (39, 17.307)
  line L21 (39, 17.307) -> (39, 18.407)
  line L22 (35.75, 12.2) -> (34.95, 12.2)
  line L23 (34.95, 12.2) -> (34.95, 11.1)
  line L24 (34.95, 11.1) -> (35.75, 11.1)
  line L25 (35.75, 11.1) -> (35.75, 12.2)
  line L26 (39, 12.2) -> (39.8, 12.2)
  line L27 (39.8, 12.2) -> (39.8, 11.1)
  line L28 (39.8, 11.1) -> (39, 11.1)
  line L29 (39, 11.1) -> (39, 12.2)
  point P0 (0, 0)
  dimension "d213" = 0.8
  dimension "d214" = 1.1
  dimension "d215" = 0.8
  dimension "d216" = 1.1
  dimension "d217" = 1.1
  constraints: 48 end point, 12 parallel, 6 horizontal, 6 perpendicular, 6 point on line
  measures "d213" distance of L8.end L7.end
  measures "d214" distance of L7.end L6.end
  measures "d215" distance of L11.end L12.end
  measures "d216" distance of L15.end L14.end
  measures "d217" distance of L23.end L22.end
extrude "Extrusion31" add sketch "Sketch32" along normal blind 0.1
equation "\"d55\" = d227"
body "Solid1"
